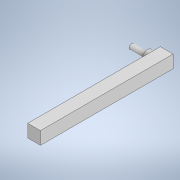
# Autodesk Inventor part: stav
Saved by Autodesk Inventor 2021 (Build 250183000, 183)
## iProperties
Created: 2021-02-09
Part Number: stav
Material: Generic
Document SubType Name: Modeling
Designer: marcu
Density: 1 g/cm^3
Appearance: Default
Author: marcu
Autodesk Inventor part; units mm, degrees
ref_plane "YZ Plane" through (0, 0, 0) normal (1, 0, 0) x (0, 1, 0)
ref_plane "XZ Plane" through (0, 0, 0) normal (0, 1, 0) x (-1, 0, 0)
ref_plane "XY Plane" through (0, 0, 0) normal (0, 0, 1) x (1, 0, 0)
sketch "Sketch1" plane through (0, 0, 0) normal (0, 0, 1) x (1, 0, 0)
  line L0 (-12.25, 12.25) -> (12.25, 12.25)
  line L1 (12.25, 12.25) -> (12.25, -12.25)
  line L2 (12.25, -12.25) -> (-12.25, -12.25)
  line L3 (-12.25, -12.25) -> (-12.25, 12.25)
  point P0 (0, 0)
  dimension "d17" = 24.5
  dimension "d18" = 24.5
  dimension "d19" = 12.25
  dimension "d20" = 12.25
  constraints: 8 end point, 2 parallel, 1 horizontal, 1 perpendicular
  measures "d17" distance of L1.end L2.end
  measures "d18" distance of L0.end L1.end
  measures "d19" distance from line of L0 point (0, 0)
  measures "d20" distance from line of L3 point (0, 0)
extrude "Extrusion1" add sketch "Sketch1" along normal blind 255
sketch "Sketch4" plane through (-12.25, -12.25, 0) normal (-1, 0, 0) x (0, 0, 1)
  circle A0 centre (15, 12.25) radius 10
  point P0 (0, 12.25)
  dimension "d22" = 20
  dimension "d23" = 15
  constraints: 1 centre point
  measures "d22" diameter of A0
  measures "d23" distance of point (0, 12.25) A0.centre
extrude "Extrusion4" add sketch "Sketch4" along normal blind 10
sketch "Sketch5" plane through (-22.25, 0, 15) normal (-1, 0, 0) x (0, 0, 1)
  circle A0 centre (0, 0) radius 5
  point P0 (-15, 0)
  dimension "d26" = 10
  constraints: 1 centre point
  measures "d26" diameter of A0
extrude "Extrusion5" add sketch "Sketch5" along normal blind 30
equation "\"d19\" = 0.5 * d18"
equation "\"d20\" = 0.5 * d17"
body "Solid1"
